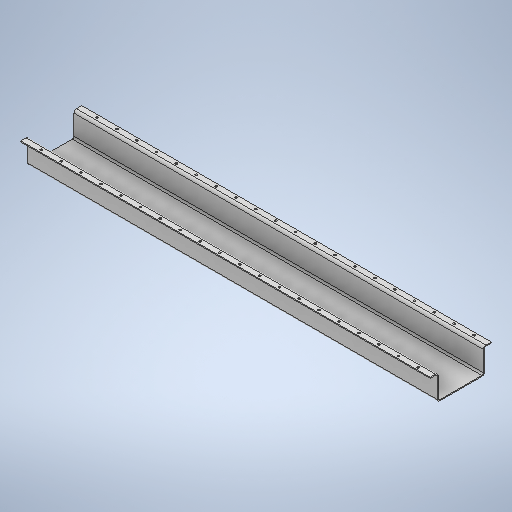
# Autodesk Inventor part: MSC 081 pillar 1_CPY
Saved by Autodesk Inventor 2025 (Build 290162010, 162A)
## iProperties
Created: 2024-06-25
Part Number: MSC 081 pillar 1_CPY
Material: Stainless Steel
Document SubType Name: Sheet Metal
Designer: admin
Density: 8 g/cm^3
Sheet Metal Rule: AISI304 3mm Die 32
Appearance: Default
Author: admin
Autodesk Inventor part; units mm, degrees
ref_plane "YZ Plane" through (0, 0, 0) normal (1, 0, 0) x (0, 1, 0)
ref_plane "XZ Plane" through (0, 0, 0) normal (0, 1, 0) x (-1, 0, 0)
ref_plane "XY Plane" through (0, 0, 0) normal (0, 0, 1) x (1, 0, 0)
sketch3d "3D Sketch1"
sketch "Sketch1" plane through (0, 0, 0) normal (0, 0, 1) x (1, 0, 0)
  line L0 (-650, 75) -> (650, 75)
  line L1 (650, 75) -> (650, -75)
  line L2 (650, -75) -> (-650, -75)
  line L3 (-650, -75) -> (-650, 75)
  line L4 (-650, 75) -> (650, -75) construction
  line L5 (650, 75) -> (-650, -75) construction
  point P0 (0, 0)
  dimension "d5" = 1300
  dimension "d30" = 150
  measures "d5" distance of L1.end L2.end
  measures "d30" distance of L2.end L0.start
extrude "Plate1" add sketch "Sketch1" along normal blind 3
sketch "Sketch6" plane through (650, -72, 0) normal (0, -1, 0) x (1, 0, 0)
  line L0 (-1300, 0) -> (0, 0)
  line L1 (0, 0) -> (0, 80)
  line L2 (0, 80) -> (-1300, 80)
  line L3 (-1300, 80) -> (-1300, 0)
  constraints: 6 end point, 1 horizontal, 1 perpendicular, 1 vertical
edge flange "Flange4" height 80 angle 90 thickness 3 bend radius 5 thickness toward (0, -1, 0) relief round relief width 3 relief depth 1.5 corner gap 5 corner form 0 edges at (0, -75, 3) (0, 75, 3) wall of the first edge with corners at (-650, -72, 0) (650, -72, 0) (650, -72, 80) (-650, -72, 80)
bend "Bend4"
corner "Corner4"
sketch "Sketch9" plane through (-650, -72, 77) normal (0, 0, 1) x (1, 0, 0)
  line L0 (1300, 0) -> (0, 0)
  line L1 (0, 0) -> (0, -25)
  line L2 (0, -25) -> (1300, -25)
  line L3 (1300, -25) -> (1300, 0)
  constraints: 6 end point, 1 horizontal, 1 perpendicular, 1 vertical
edge flange "Flange5" height 22 angle 90 thickness 3 bend radius 5 thickness toward (0, 0, 1) relief round relief width 3 relief depth 1.5 edges at (0, -75, 80) wall of the first edge with corners at (650, -72, 77) (-650, -72, 77) (-650, -97, 77) (650, -97, 77)
bend "Bend5"
corner "Corner5"
sketch "Sketch10" plane through (650, 72, 77) normal (0, 0, 1) x (1, 0, 0)
  line L0 (-1300, 0) -> (0, 0)
  line L1 (0, 0) -> (0, 25)
  line L2 (0, 25) -> (-1300, 25)
  line L3 (-1300, 25) -> (-1300, 0)
  constraints: 6 end point, 1 horizontal, 1 perpendicular, 1 vertical
edge flange "Flange6" height 22 angle 90 thickness 3 bend radius 5 thickness toward (0, 0, 1) relief round relief width 3 relief depth 1.5 edges at (0, 75, 80) wall of the first edge with corners at (-650, 72, 77) (650, 72, 77) (650, 97, 77) (-650, 97, 77)
bend "Bend6"
corner "Corner6"
sketch "Sketch11" plane through (-650, -97, 80) normal (0, 0, 1) x (1, 0, 0)
  circle A0 centre (1254, 8.5) radius 3.5
  line L0 (1300, 17) -> (1300, 0) projected
  point P0 (650, 97)
  point P1 (1300, 8.5)
  point P2 (1300, 8.5)
  dimension "d101" = 46
  dimension "d102" = 7
  constraints: 2 midpoint, 1 centre point, 1 horizontal alignment
  measures "d101" distance of point (1300, 8.5) A0.centre
  measures "d102" diameter of A0
extrude "Cut1" cut sketch "Sketch11" against normal blind 3
pattern_linear "Rectangular Pattern2" count 20 spacing 63 along (-1, 0, 0) of "Cut1"
mirror "Mirror2" about plane through (0, 0, 0) normal (0, 1, 0) of "Cut1", "Rectangular Pattern2"
equation "\"d112\" = Thickness"
equation "\"d6\" = Thickness"
equation "\"d60\" = BendReliefWidth"
equation "\"d61\" = BendReliefDepth"
equation "\"d62\" = MinimumRemnant"
equation "\"d63\" = TransitionRadius"
equation "\"d66\" = BendRadius"
equation "\"d67\" = CornerReliefSize"
equation "\"d68\" = GapSize"
equation "\"d69\" = JacobiRadiusSize"
equation "\"d81\" = BendReliefWidth"
equation "\"d82\" = BendReliefDepth"
equation "\"d83\" = MinimumRemnant"
equation "\"d84\" = TransitionRadius"
equation "\"d87\" = BendRadius"
equation "\"d88\" = CornerReliefSize"
equation "\"d89\" = GapSize"
equation "\"d90\" = JacobiRadiusSize"
equation "\"d91\" = BendReliefWidth"
equation "\"d92\" = BendReliefDepth"
equation "\"d93\" = MinimumRemnant"
equation "\"d94\" = TransitionRadius"
equation "\"d97\" = BendRadius"
equation "\"d98\" = CornerReliefSize"
equation "\"d99\" = GapSize"
equation "\"d100\" = JacobiRadiusSize"
equation "\"BendReliefWidth\" = Thickness"
equation "\"BendReliefDepth\" = 0.5 * Thickness"
equation "\"CornerReliefSize\" = 4 * Thickness"
equation "\"MinimumRemnant\" = 2 * Thickness"
equation "\"TransitionRadius\" = BendRadius"
equation "\"JacobiRadiusSize\" = BendRadius"
equation "\"GapSize\" = Thickness"
equation "\"Thickness\" = 3"
equation "\"BendRadius\" = 5"
body "Solid1"
